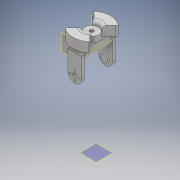
# Autodesk Inventor part: middle_joint_microservo_metalico
Saved by Autodesk Inventor 2018 (Build 220112000, 112)
## iProperties
Created: 2018-02-12
Part Number: middle_joint_microservo_metalico
Material: Generic
Document SubType Name: Modeling
Designer: Bardo91
Density: 1 g/cm^3
Appearance: Default
Author: Bardo91
Autodesk Inventor part; units mm, degrees
ref_plane "YZ Plane" through (0, 0, 0) normal (1, 0, 0) x (0, 1, 0)
ref_plane "XZ Plane" through (0, 0, 0) normal (0, 1, 0) x (-1, 0, 0)
ref_plane "XY Plane" through (0, 0, 0) normal (0, 0, 1) x (1, 0, 0)
sketch "Sketch1" plane through (0, 0, 0) normal (0, 0, 1) x (1, 0, 0)
  line L0 (0, 0) -> (18, 0)
  line L1 (18, 0) -> (18, 32)
  line L2 (18, 32) -> (0, 32)
  line L3 (0, 32) -> (0, 0)
  dimension "d0" = 18
  dimension "d1" = 32
  constraints: 8 end point, 2 perpendicular, 1 horizontal, 1 vertical
  measures "d0" distance of L0.start L0.end
  measures "d1" distance of L0.end L1.end
extrude "base" add sketch "Sketch1" along normal blind 15
ref_plane "Work Plane1" through (9, 22, -120) normal (0, 0, -1) x (-1, 0, 0)
ref_plane "Work Plane2" through (0, 0, 10) normal (0, 0, -1) x (-1, 0, 0)
sketch "Sketch12" plane through (0, 0, 10) normal (0, 0, -1) x (-1, 0, 0)
  line L0 (0, 0) -> (-18, 0) projected
  line L1 (-18, 0) -> (-18, -4)
  line L2 (-18, -4) -> (0, -4)
  line L3 (0, -4) -> (0, 0)
  line L4 (0, 0) -> (0, -4)
  line L5 (0, 0) -> (-18, 0)
  line L6 (-18, 32) -> (0, 32) projected
  line L7 (-18, 32) -> (0, 32)
  line L8 (0, 32) -> (0, 36)
  line L9 (0, 36) -> (-18, 36)
  line L10 (-18, 36) -> (-18, 32)
  dimension "d64" = 4
  dimension "d65" = 4
  constraints: 18 end point, 4 perpendicular, 3 collinear, 2 point on line, 1 vertical
  measures "d64" distance of L0.end L1.end
  measures "d65" distance of L6.end L8.end
extrude "connector_prev_servo" add sketch "Sketch12" along normal blind 36
fillet "Fillet3" radius 9 4 edges at (18, 34, -26) (0, 34, -26) (0, -2, -26) (18, -2, -26)
ref_plane "Work Plane6" through (0, -4, 10) normal (0, -1, 0) x (1, 0, 0)
sketch "Sketch13" plane through (0, -4, 10) normal (0, -1, 0) x (1, 0, 0)
  arc A0 (0, -27) -> (18, -27) centre (9, -27) ccw projected
  circle A1 centre (9, -27) radius 2.75
  line L0 (9, -27) -> (15, -27)
  circle A2 centre (15, -27) radius 1
  circle A3 centre (9, -21) radius 1
  circle A4 centre (3, -27) radius 1
  circle A5 centre (9, -33) radius 1
  point P0 (0, -10)
  dimension "d72" = 5.5
  dimension "d73" = 6
  dimension "d74" = 2
  dimension "d77" = 360
  constraints: 5 centre point, 2 coincident, 2 end point, 1 horizontal, 9 other
  measures "d72" diameter of A1
  measures "d73" distance of L0.start L0.end
  measures "d74" diameter of A2
extrude "screw_holes" cut sketch "Sketch13" against normal up to surface (4 mm away)
fillet "Fillet4" radius 9 2 edges at (18, 16, 0) (0, 16, 0)
ref_plane "Work Plane7" through (0, 36, 10) normal (0, 1, 0) x (1, 0, 0)
sketch "Sketch14" plane through (0, 36, 10) normal (0, 1, 0) x (1, 0, 0)
  arc A0 (18, 27) -> (0, 27) centre (9, 27) ccw projected
  circle A1 centre (9, 27) radius 5.25
  point P0 (0, 10)
  dimension "d82" = 10.5
  constraints: 1 centre point, 1 coincident
  measures "d82" diameter of A1
extrude "Extrusion14" add sketch "Sketch14" against normal blind 6
sketch "Sketch26" plane through (0, 0, 15) normal (0, 0, 1) x (1, 0, 0)
  line L0 (18, 32) -> (0, 32) projected
  line L1 (9, 32) -> (9, 0)
  line L2 (8, -4) -> (8, 0) projected
  arc A0 (-8, -2.3303) -> (26, -2.3303) centre (9, 16) ccw
  arc A1 (26, 34.3303) -> (-8, 34.3303) centre (9, 16) ccw
  arc A2 (-8, -2.3303) -> (2.88, 9.4011) centre (-16, 16) ccw
  arc A3 (2.88, 22.5989) -> (-8, 34.3303) centre (-16, 16) ccw
  arc A4 (26, 34.3303) -> (15.12, 22.5989) centre (34, 16) ccw
  arc A5 (15.12, 9.4011) -> (26, -2.3303) centre (34, 16) ccw
  arc A6 (2.88, 22.5989) -> (2.88, 9.4011) centre (9, 16) ccw
  arc A7 (15.12, 9.4011) -> (15.12, 22.5989) centre (9, 16) ccw
  point P0 (0, 0)
  dimension "d167" = 25
  constraints: 16 point on circle, 8 centre point, 2 end point, 2 midpoint, 1 coincident, 1 parallel
  measures "d167" radius of A1
extrude "Extrusion26" add sketch "Sketch26" along normal blind 13
fillet "Fillet6" radius 2 4 edges at (26, -2.3303, 21.5) (26, 34.3303, 21.5) (-8, 34.3303, 21.5) (-8, -2.3303, 21.5)
sketch "Sketch27" plane through (0, 0, 28) normal (0, 0, 1) x (1, 0, 0)
  arc A0 (0, 16) -> (2.88, 9.4011) centre (9, 16) ccw projected
  circle A1 centre (9, 16) radius 9
  point P0 (0, 0)
  constraints: 1 centre point, 1 coincident
extrude "Extrusion27" cut sketch "Sketch27" against normal blind 5
fillet "Fillet7" radius 5 2 edges at (9, 7, 28) (9, 25, 28)
sketch "Sketch28" plane through (0, 0, 23) normal (0, 0, 1) x (1, 0, 0)
  arc A0 (0, 16) -> (2.88, 9.4011) centre (9, 16) ccw projected
  circle A1 centre (9, 16) radius 2.5
  point P0 (0, 0)
  dimension "d164" = 5
  constraints: 1 centre point, 1 coincident
  measures "d164" diameter of A1
extrude "Extrusion28" cut sketch "Sketch28" against normal through all
sketch "Sketch29" plane through (0, 0, 28) normal (0, 0, 1) x (1, 0, 0)
  circle A0 centre (9, 16) radius 2.5 projected
  circle A1 centre (9, 16) radius 24.85
  circle A2 centre (9, 16) radius 30
  point P0 (0, 0)
  dimension "d168" = 49.7
  dimension "d169" = 60
  constraints: 2 centre point, 2 coincident
  measures "d168" diameter of A1
  measures "d169" diameter of A2
extrude "Extrusion29" cut sketch "Sketch29" against normal up to surface (18 mm away) contours A2
move faces "Desplazar1" translate (0, -2.5, 0) faces at (9.0402, -4, 3.3309) (13.2838, 0, -8.2123)
move faces "Desplazar2" translate (0, 2.5, 0) faces at (2.8196, 32, -9.5184) (6, 36, 1) (10.6257, 30, -18.4402)
sketch "Boceto30" plane through (9, 32.5, -17) normal (0, -1, 0) x (1, 0, 0)
  circle A0 centre (0, 0) radius 5.25
  circle A1 centre (0, 0) radius 4.75
  point P0 (-9, 17)
  dimension "d178" = 9.5
  constraints: 2 centre point, 1 coincident
  measures "d178" diameter of A1
extrude "Extrusión30" cut sketch "Boceto30" against normal blind 2
body "Solid1"
